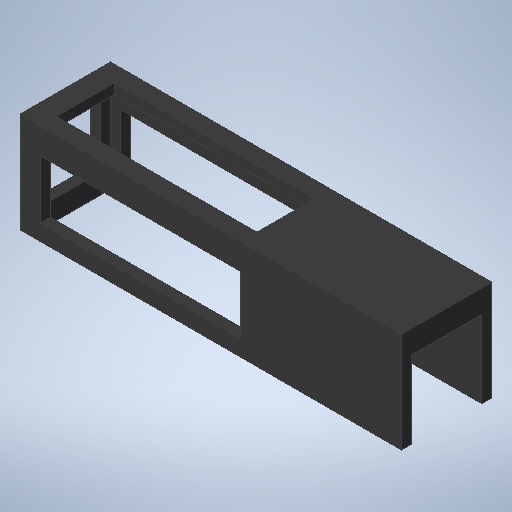
# Autodesk Inventor part: PipetteStand
Saved by Autodesk Inventor 2025.1 (Build 291241000, 241)
## iProperties
Created: 2024-11-06
Part Number: PipetteStand
Material: Generic
Document SubType Name: Modeling
Designer: 13156
Density: 1 g/cm^3
Appearance: Default
Author: 13156
Autodesk Inventor part; units mm, degrees
ref_plane "YZ Plane" through (0, 0, 0) normal (1, 0, 0) x (0, 1, 0)
ref_plane "XZ Plane" through (0, 0, 0) normal (0, 1, 0) x (-1, 0, 0)
ref_plane "XY Plane" through (0, 0, 0) normal (0, 0, 1) x (1, 0, 0)
sketch "Sketch2" plane through (0, 0, 0) normal (1, 0, 0) x (0, 1, 0)
  line L0 (25, 22.5) -> (-25, 22.5)
  line L1 (-25, 22.5) -> (-25, -22.5)
  line L2 (-25, -22.5) -> (25, -22.5)
  line L3 (25, -22.5) -> (25, 22.5)
  point P0 (0, 0)
  point P1 (-25, 0)
  point P2 (25, 0)
  dimension "d0" = 45
  dimension "d1" = 50
  dimension "d2" = 25
  dimension "d3" = 22.5
  constraints: 8 end point, 2 midpoint, 2 parallel, 1 horizontal, 1 perpendicular
  measures "d0" distance between parallel lines of L2 L0
  measures "d1" distance from line of point (-25, 0) L3
  measures "d2" distance of point (0, 0) point (25, 0)
  measures "d3" distance from line of point (0, 0) L2
extrude "Extrusion1" add sketch "Sketch2" along normal blind 125.1
sketch "Sketch3" plane through (0, -25, -22.5) normal (0, -1, 0) x (1, 0, 0)
  line L0 (125.1, 45) -> (125.1, 0) projected
  line L1 (125.1, 40) -> (5, 40)
  line L2 (5, 40) -> (5, 5)
  line L3 (5, 5) -> (125.1, 5)
  line L4 (125.1, 5) -> (125.1, 40)
  line L5 (0, 45) -> (0, 0) projected
  line L6 (0, 0) -> (125.1, 0) projected
  line L7 (0, 45) -> (125.1, 45) projected
  point P0 (0, 22.5)
  point P1 (125.1, 5)
  dimension "d6" = 5
  dimension "d7" = 35
  dimension "d8" = 5
  dimension "d45" = 5
  constraints: 8 end point, 2 parallel, 1 horizontal, 1 perpendicular, 1 point on line
  measures "d6" distance between parallel lines of L5 L2
  measures "d7" distance between parallel lines of L3 L1
  measures "d8" distance between parallel lines of L6 L3
  measures "d45" distance between parallel lines of L7 L1
extrude "Extrusion2" cut sketch "Sketch3" against normal blind 38.5 contours L0 L3 L2 L1
sketch "Sketch4" plane through (0, 0, 0) normal (-1, 0, 0) x (0, 0, 1)
  line L0 (22.5, -25) -> (17.5, -25) projected
  line L1 (-22.5, 25) -> (22.5, 25) projected
  line L2 (22.5, -25) -> (-22.5, -25)
  line L3 (-22.5, -25) -> (-22.5, 25)
  line L4 (-22.5, 25) -> (22.5, 25)
  line L5 (22.5, 25) -> (22.5, -25)
  line L6 (17.5, -25) -> (-17.5, -25)
  line L7 (-17.5, -25) -> (-17.5, 20)
  line L8 (-17.5, 20) -> (17.5, 20)
  line L9 (17.5, 20) -> (17.5, -25)
  point P0 (0, 0)
  point P1 (-17.5, -25)
  dimension "d11" = 5
  dimension "d12" = 5
  dimension "d13" = 5
  constraints: 16 end point, 4 parallel, 2 horizontal, 2 perpendicular, 1 point on line
  measures "d11" distance between parallel lines of L5 L9
  measures "d12" distance between parallel lines of L3 L7
  measures "d13" distance between parallel lines of L1 L8
extrude "Extrusion3" add sketch "Sketch4" along normal blind 120 contours L0 L9 L8 L7 L2 L3 L1 L5
sketch "Sketch5" plane through (0, 0, 0) normal (-1, 0, 0) x (0, 0, 1)
  line L0 (17.5, -25) -> (-17.5, -25) projected
  line L1 (11, -25) -> (-11, -25)
  line L2 (-11, -25) -> (-11, 8.5)
  line L3 (-11, 8.5) -> (11, 8.5)
  line L4 (11, 8.5) -> (11, -25)
  line L5 (17.5, 20) -> (17.5, -25) projected
  line L6 (-17.5, -25) -> (-17.5, 20) projected
  line L7 (-17.5, 20) -> (17.5, 20) projected
  point P0 (0, 0)
  dimension "d16" = 6.5
  dimension "d17" = 6.5
  dimension "d18" = 11.5
  constraints: 8 end point, 2 parallel, 1 horizontal, 1 perpendicular, 1 point on line
  measures "d16" distance between parallel lines of L5 L4
  measures "d17" distance between parallel lines of L6 L2
  measures "d18" distance between parallel lines of L7 L3
extrude "Extrusion4" cut sketch "Sketch5" against normal blind 5 contours L0 L2 L3 L4
sketch "Sketch6" plane through (-120, 0, 0) normal (-1, 0, 0) x (0, 0, 1)
  line L0 (-22.5, 25) -> (22.5, 25) projected
  line L1 (-17.5, -25) -> (-22.5, -25) projected
  line L2 (22.5, 25) -> (-22.5, 25)
  line L3 (-22.5, 25) -> (-22.5, -25)
  line L4 (-22.5, -25) -> (22.5, -25)
  line L5 (22.5, -25) -> (22.5, 25)
  point P0 (0, 0)
  constraints: 8 end point, 2 parallel, 1 horizontal, 1 perpendicular
extrude "Extrusion5" add sketch "Sketch6" against normal blind 5
sketch "Sketch7" plane through (125.1, 0, 0) normal (1, 0, 0) x (0, 0, -1)
  line L0 (22.5, 25) -> (-22.5, 25) projected
  line L1 (22.5, -25) -> (22.5, 25) projected
  line L2 (-22.5, 25) -> (22.5, 25)
  line L3 (22.5, 25) -> (22.5, -25)
  line L4 (22.5, -25) -> (-22.5, -25)
  line L5 (-22.5, -25) -> (-22.5, 25)
  point P0 (0, 0)
  constraints: 8 end point, 2 parallel, 1 horizontal, 1 perpendicular
extrude "Extrusion6" cut sketch "Sketch7" against normal blind 55
sketch "Sketch9" plane through (-120, -25, 22.5) normal (0, 0, 1) x (1, 0, 0)
  line L0 (110, 37) -> (10, 37)
  line L1 (10, 37) -> (10, 8)
  line L2 (10, 8) -> (110, 8)
  line L3 (110, 8) -> (110, 37)
  line L4 (0, 0) -> (0, 50) projected
  line L5 (190.1, 0) -> (0, 0) projected
  line L6 (120, 45) -> (5, 45) projected
  point P0 (120, 25)
  point P1 (120, 0)
  dimension "d27" = 10
  dimension "d28" = 10
  dimension "d29" = 8
  dimension "d30" = 8
  constraints: 8 end point, 2 parallel, 1 horizontal, 1 perpendicular
  measures "d27" distance between parallel lines of L4 L1
  measures "d28" distance from line of point (120, 0) L3
  measures "d29" distance between parallel lines of L5 L2
  measures "d30" distance between parallel lines of L6 L0
extrude "Extrusion8" cut sketch "Sketch9" against normal blind 77.225
sketch "Sketch10" plane through (0, 20, -17.5) normal (0, -1, 0) x (1, 0, 0)
  line L0 (-10, 32) -> (-110, 32)
  line L1 (-110, 32) -> (-110, 3)
  line L2 (-110, 3) -> (-10, 3)
  line L3 (-10, 3) -> (-10, 32)
  line L4 (-120, -5) -> (-120, 40) projected
  line L5 (0, 35) -> (0, 28.5) projected
  line L6 (-120, -5) -> (70.1, -5) projected
  line L7 (70.1, 40) -> (-120, 40) projected
  point P0 (0, 17.5)
  point P1 (0, 31.75)
  dimension "d33" = 10
  dimension "d34" = 10
  dimension "d35" = 8
  dimension "d36" = 8
  constraints: 8 end point, 2 parallel, 1 horizontal, 1 midpoint, 1 perpendicular
  measures "d33" distance between parallel lines of L4 L1
  measures "d34" distance from line of point (0, 31.75) L3
  measures "d35" distance between parallel lines of L6 L2
  measures "d36" distance between parallel lines of L7 L0
extrude "Extrusion9" cut sketch "Sketch10" against normal blind 77.225
sketch "Sketch11" plane through (-120, 0, 0) normal (-1, 0, 0) x (0, 0, 1)
  line L0 (12.5, -15) -> (-12.5, -15)
  line L1 (-12.5, -15) -> (-12.5, 15)
  line L2 (-12.5, 15) -> (12.5, 15)
  line L3 (12.5, 15) -> (12.5, -15)
  line L4 (-22.5, -25) -> (22.5, -25) projected
  line L5 (-22.5, 25) -> (-22.5, -25) projected
  line L6 (22.5, 25) -> (-22.5, 25) projected
  line L7 (22.5, -25) -> (22.5, 25) projected
  point P0 (0, 0)
  dimension "d39" = 10
  dimension "d40" = 10
  dimension "d41" = 10
  dimension "d42" = 10
  constraints: 8 end point, 2 parallel, 1 horizontal, 1 perpendicular
  measures "d39" distance between parallel lines of L4 L0
  measures "d40" distance between parallel lines of L5 L1
  measures "d41" distance between parallel lines of L6 L2
  measures "d42" distance between parallel lines of L7 L3
extrude "Extrusion10" cut sketch "Sketch11" against normal blind 16.9 contours L0 L1 L2 L3
body "Solid1"
